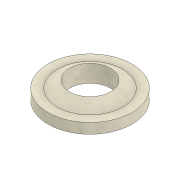
# Autodesk Inventor part: 胶垫
Saved by Autodesk Inventor 2022 (Build 260153000, 153)
## iProperties
Created: 2023-03-14
Part Number: 胶垫
Material: 亚麻布，米色
Document SubType Name: Modeling
Designer: Lzy18
Density: 0.152 g/cm^3
Appearance: 亚麻布 - 米色
Author: Lzy18
Autodesk Inventor part; units mm, degrees
ref_plane "YZ Plane" through (0, 0, 0) normal (1, 0, 0) x (0, 1, 0)
ref_plane "XZ Plane" through (0, 0, 0) normal (0, 1, 0) x (-1, 0, 0)
ref_plane "XY Plane" through (0, 0, 0) normal (0, 0, 1) x (1, 0, 0)
sketch "草图1" plane through (0, 0, 0) normal (0, 0, 1) x (1, 0, 0)
  line L0 (-10, 8.4641) -> (-10, 0)
  line L1 (-20.5, 5) -> (-20.5, 0)
  line L2 (-20.5, 0) -> (-10, 0)
  line L3 (-20.5, 5) -> (-16, 5)
  line L4 (-16, 5) -> (-10, 8.4641)
  line L5 (0, -1.6928) -> (0, 10.1569) projected
  point P0 (0, 0)
  dimension "d0" = 10
  dimension "d2" = 5
  dimension "d3" = 16
  dimension "d4" = 20.5
  dimension "d5" = 60
  constraints: 10 end point, 2 horizontal, 2 vertical
  measures "d0" distance from line of point (0, 0) L0
  measures "d2" distance of L1.start L1.end
  measures "d3" horizontal distance of point (0, 0) L3.end
  measures "d4" distance of point (0, 0) L1.end
  measures "d5" angle of L0 L4
revolve "旋转1" add sketch "草图1" angle 360 about axis through (0, -10, 0) along (0, 1, 0)
